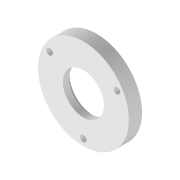
# Autodesk Inventor part: 50_ETL_Base_layer1_v0
Saved by Autodesk Inventor 2022 (Build 260153000, 153)
## iProperties
Created: 2021-12-31
Part Number: 50_ETL_Base_layer1_v0
Material: Generisch
Document SubType Name: Modeling
Designer: diederichbenedict
Density: 1 g/cm^3
Appearance: Vorgabe
Author: diederichbenedict
Autodesk Inventor part; units mm, degrees
ref_plane "YZ Plane" through (0, 0, 0) normal (1, 0, 0) x (0, 1, 0)
ref_plane "XZ Plane" through (0, 0, 0) normal (0, 1, 0) x (-1, 0, 0)
ref_plane "XY Plane" through (0, 0, 0) normal (0, 0, 1) x (1, 0, 0)
sketch "Skizze1" plane through (0, 0, 0) normal (0, 1, 0) x (-1, 0, 0)
  line L0 (-6.65, -5) -> (-6.65, 0)
  line L1 (31.95, 0) -> (-6.65, 0) projected
  line L2 (25.15, 0.6) -> (0.15, 0.6) projected
  line L3 (0.15, 0) -> (0.15, 0.6)
  line L4 (25.65, 5.6) -> (-0.35, 5.6) projected
  line L5 (-6.65, 0) -> (-0.0746, 0)
  line L6 (-0.0746, 0) -> (-0.0746, 0.397)
  line L7 (-0.0746, 0.397) -> (3.1743, 0.397) construction
  line L8 (3.9432, 5.6) -> (-6.65, 5.6)
  line L9 (-6.65, 5.6) -> (-6.65, 0)
  line L10 (0.15, 2.6301) -> (2.65, 2.6301)
  line L11 (2.65, 2.6301) -> (2.65, 0.1301)
  line L12 (2.65, 0.1301) -> (0.15, 0.1301)
  line L13 (0.15, 0.1301) -> (0.15, 2.6301)
  line L14 (0.15, 2.6301) -> (2.65, 0.1301) construction
  line L15 (2.65, 2.6301) -> (0.15, 0.1301) construction
  line L16 (2.65, 1.4705) -> (3.9432, 2.9441)
  line L17 (3.9432, 2.9441) -> (3.9432, 5.6)
  line L18 (12.65, 7.6215) -> (12.65, -1.0202)
  line L19 (4.6015, 2.505) -> (4.6015, 3.505)
  line L20 (20.6985, 2.505) -> (20.6985, 3.505)
  line L21 (-0.0746, 0.397) -> (0.15, 0.397)
  point P0 (0, 0)
  point P1 (1.4, 1.3801)
  point P2 (0.15, 0.397)
  point P3 (2.65, 0.6)
  point P4 (0.15, 0.1301)
  dimension "d0" = 2.5
  dimension "d1" = 2.5
  dimension "d3" = 16.0971
  dimension "d4" = 8.0485
  dimension "d5" = 11.25
  constraints: 38 end point, 5 point on line, 5 vertical, 4 perpendicular, 3 parallel, 2 horizontal, 2 midpoint, 1 coincident, 7 other
  measures "d0" distance of L11.end L12.end
  measures "d1" distance of L10.end L11.end
  measures "d3" distance between parallel lines of L20 L19
  measures "d4" distance between parallel lines of L19 L18
  measures "d5" distance from line of L18 point (1.4, 1.38)
revolve "Umdrehung1" add sketch "Skizze1" angle 360 about axis through (-12.65, 0, 7.6215) along (0, 0, -1) contours L1 L6 L21 L3 | L1 L9 L8 L4 L17 L16 L11 L10 L13 L3 L21 L6
sketch "Skizze2" plane through (-12.65, 0, 5.6) normal (0, 0, 1) x (1, 0, 0)
  circle A0 centre (14.2894, 8.25) radius 1.4 projected
  circle A1 centre (-14.2894, 8.25) radius 1.4 projected
  arc A2 (-6.25, 7.8062) -> (6.25, 7.8062) centre (0, 0) ccw projected
  circle A3 centre (0, -16.5) radius 1.4 projected
  point P0 (12.65, 0)
extrude "Extrusion1" cut sketch "Skizze2" against normal blind 10
equation "\"d4\" = 0.5 * d3"
